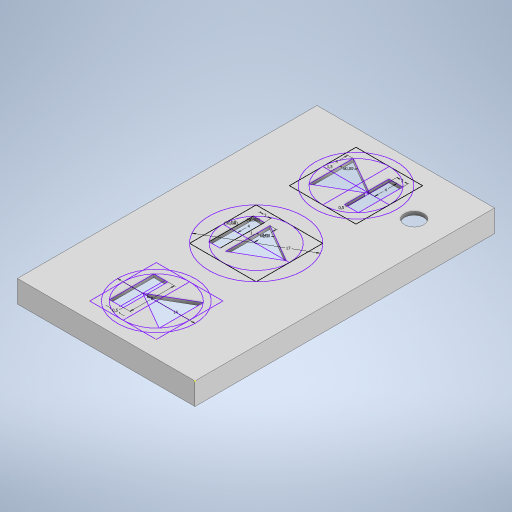
# Autodesk Inventor part: button_top
Saved by Autodesk Inventor 2024.3 (Build 283343000, 343)
## iProperties
Created: 2025-07-27
Part Number: button_top
Material: Ogólny
Document SubType Name: Modeling
Designer: User
Density: 1 g/cm^3
Appearance: Domyślna
Author: User
Autodesk Inventor part; units mm, degrees
ref_plane "YZ Plane" through (0, 0, 0) normal (1, 0, 0) x (0, 1, 0)
ref_plane "XZ Plane" through (0, 0, 0) normal (0, 1, 0) x (-1, 0, 0)
ref_plane "XY Plane" through (0, 0, 0) normal (0, 0, 1) x (1, 0, 0)
sketch "Szkic1" plane through (0, 0, 0) normal (0, 1, 0) x (-1, 0, 0)
  line L0 (0, 0) -> (32, 0)
  line L1 (32, 0) -> (32, -54)
  line L2 (32, -54) -> (0, -54)
  line L3 (0, -54) -> (0, 0)
  line L4 (32, -54) -> (32, -36)
  line L5 (32, -36) -> (0, -36)
  line L6 (32, 0) -> (32, -18)
  line L7 (32, -18) -> (0, -18)
  line L8 (32, -18) -> (32, -16)
  line L9 (32, -18) -> (32, -20)
  line L10 (32, 0) -> (32, -2)
  line L11 (32, 0) -> (32, -2)
  line L12 (32, -2) -> (0, -2)
  line L13 (0, -2) -> (0, 0)
  line L14 (0, 0) -> (32, 0)
  line L15 (32, -16) -> (32, -20)
  line L16 (32, -20) -> (0, -20)
  line L17 (0, -20) -> (0, -16)
  line L18 (0, -16) -> (32, -16)
  line L19 (32, 0) -> (32, -20)
  line L20 (32, -20) -> (30, -20)
  line L21 (30, -20) -> (30, 0)
  line L22 (30, 0) -> (32, 0)
  line L23 (0, 0) -> (0, -20)
  line L24 (0, -20) -> (2, -20)
  line L25 (2, -20) -> (2, 0)
  line L26 (2, 0) -> (0, 0)
  line L27 (16, -54) -> (16, -45)
  line L28 (16, -54) -> (25, -54) construction
  circle A0 centre (16, -45) radius 1.5
  circle A1 centre (16, -27) radius 1.5
  circle A2 centre (16, -9) radius 1.5
  line L29 (32, -20) -> (0, -20)
  line L30 (30, -38) -> (30, -18)
  line L31 (0, -34) -> (32, -34)
  line L32 (2, -38) -> (2, -18)
  line L33 (32, -38) -> (0, -38)
  line L34 (30, -56) -> (30, -36)
  line L35 (0, -52) -> (32, -52)
  line L36 (2, -56) -> (2, -36)
  line L37 (30, -2) -> (30, -1)
  line L38 (2, -2) -> (2, -1)
  line L39 (30, -2) -> (31, -2)
  line L40 (2, -16) -> (2, -17)
  line L41 (2, -17) -> (1, -17)
  line L42 (1, -17) -> (31, -17)
  line L43 (31, -17) -> (31, -1)
  line L44 (31, -1) -> (1, -1)
  line L45 (1, -1) -> (1, -17)
  line L46 (31, -35) -> (31, -19)
  line L47 (1, -35) -> (31, -35)
  line L48 (1, -19) -> (1, -35)
  line L49 (31, -19) -> (1, -19)
  line L50 (31, -53) -> (31, -37)
  line L51 (1, -53) -> (31, -53)
  line L52 (1, -37) -> (1, -53)
  line L53 (31, -37) -> (1, -37)
  line L54 (22, -39) -> (10, -39)
  line L55 (10, -39) -> (10, -51)
  line L56 (10, -51) -> (22, -51)
  line L57 (22, -51) -> (22, -39)
  line L58 (22, -39) -> (10, -51) construction
  line L59 (10, -39) -> (22, -51) construction
  line L60 (22, -21) -> (10, -21)
  line L61 (10, -21) -> (10, -33)
  line L62 (10, -33) -> (22, -33)
  line L63 (22, -33) -> (22, -21)
  line L64 (22, -21) -> (10, -33) construction
  line L65 (10, -21) -> (22, -33) construction
  line L66 (22, -3) -> (10, -3)
  line L67 (10, -3) -> (10, -15)
  line L68 (10, -15) -> (22, -15)
  line L69 (22, -15) -> (22, -3)
  line L70 (22, -3) -> (10, -15) construction
  line L71 (10, -3) -> (22, -15) construction
  circle A3 centre (16, -45) radius 6
  circle A4 centre (16, -27) radius 6
  circle A5 centre (16, -9) radius 6
  point P0 (30, -16)
  point P1 (30, -34)
  point P2 (2, -34)
  point P3 (30, -52)
  point P4 (2, -52)
  point P5 (16, 0)
  dimension "d0" = 32
  dimension "d1" = 54
  dimension "d13" = 18
  dimension "d14" = 18
  dimension "d15" = 2
  dimension "d16" = 2
  dimension "d17" = 2
  dimension "d18" = 2
  dimension "d19" = 2
  dimension "d20" = 9
  dimension "d21" = 90
  dimension "d22" = 3
  dimension "d25" = 18
  dimension "d32" = 18
  dimension "d39" = 1
  dimension "d40" = 1
  dimension "d41" = 1
  dimension "d42" = 1
  dimension "d43" = 1
  dimension "d48" = 18
  dimension "d53" = 12
  dimension "d54" = 12
  dimension "d55" = 12
  dimension "d56" = 12
  dimension "d57" = 12
  dimension "d58" = 12
  dimension "d59" = 3
  constraints: 144 end point, 18 parallel, 17 point on line, 13 perpendicular, 8 midpoint, 6 centre point, 6 horizontal, 5 vertical, 4 coincident, 3 collinear, 1 tangent, 44 other
  measures "d0" distance of L1.end L2.end
  measures "d1" distance of L0.end L1.end
  measures "d13" distance of L1.end L4.end
  measures "d14" distance of L0.end L6.end
  measures "d15" distance of L6.end L8.end
  measures "d16" distance of L6.end L9.end
  measures "d17" distance of L0.end L10.end
  measures "d18" distance of L9.end L20.end
  measures "d19" distance of L24.end L16.end
  measures "d20" distance of L27.start L27.end
  measures "d21" angle of L28 L27
  measures "d22" diameter of A0
  measures "d25" distance of A0.centre A1.centre
  measures "d32" distance of L10.end L29.start
  measures "d39" distance of L37.start L37.end
  measures "d40" distance of L38.start L38.end
  measures "d41" distance of L37.start L39.end
  measures "d42" distance of L40.start L40.end
  measures "d43" distance of L40.end L41.end
  measures "d48" distance of L42.end L46.start
  measures "d53" distance of L56.end L55.end
  measures "d54" distance of L55.end L54.end
  measures "d55" distance of L62.end L61.end
  measures "d56" distance of L61.end L60.end
  measures "d57" distance of L68.end L67.end
  measures "d58" distance between parallel lines of L66 L68
  measures "d59" distance from line of point (16, 0) L66
extrude "Wyciągnięcie proste1" add sketch "Szkic1" along normal blind 2 contours L0 L25 L44 L45 L12 L3 | L0 L21 L44 L25 | L12 L45 L18 L3 | L0 L1 L12 L43 L44 L21 | L44 L21 L12 L25 | L25 L12 L45 L44 | L18 L45 L41 L25 L7 L3 | L12 L25 L18 L45 | L44 L43 L12 L21 | L12 L21 L18 L25 | L7 L25 L49 L48 L16 L3 | L18 L25 L41 L45 | L1 L18 L43 L12 | L12 L43 L18 L21 | L18 L21 L42 L25 | L16 L48 L31 L3 | L25 L42 L21 L7 | L7 L21 L49 L25 | L1 L7 L21 L42 L43 L18 | L18 L43 L42 L21 | L31 L48 L47 L32 L5 L3 | L48 L49 L25 L16 | L16 L32 L31 L48 | L7 L1 L16 L46 L49 L21 | L49 L21 L16 L25 | L5 L32 L53 L52 L33 L3 | L31 L32 L47 L48 | L16 L30 L31 L32 | L49 L46 L16 L21 | L1 L31 L46 L16 | L33 L52 L35 L3 | L32 L47 L30 L5 | L5 L30 L53 L32 | L31 L30 L47 L32 | L16 L46 L31 L30 | L1 L5 L30 L47 L46 L31 | L35 L52 L51 L36 L2 L3 | L52 L53 L32 L33 | L33 L36 L35 L52 | L5 L1 L33 L50 L53 L30 | L53 L30 L33 L32 | L31 L46 L47 L30 | L35 L36 L51 L52 | L33 L34 L35 L36 | L53 L50 L33 L30 | L1 L35 L50 L33 | L36 L51 L27 L2 | L35 L27 L51 L36 | L33 L50 L35 L34 | L1 L2 L34 L51 L50 L35 | L27 L51 L34 L2 | L35 L34 L51 L27 | L35 L50 L51 L34
extrude "Wyciągnięcie proste3" cut sketch "Szkic1" along normal blind 1.4 contours L44 L21 L12 L25 | L25 L12 L45 L44 | L12 L25 L18 L45 | L44 L43 L12 L21 | L12 L21 L18 L25 | L18 L25 L41 L45 | L12 L43 L18 L21 | L18 L21 L42 L25 | L18 L43 L42 L21 | L48 L49 L25 L16 | L16 L32 L31 L48 | L49 L21 L16 L25 | L31 L32 L47 L48 | L16 L30 L31 L32 | L49 L46 L16 L21 | L31 L30 L47 L32 | L16 L46 L31 L30 | L52 L53 L32 L33 | L33 L36 L35 L52 | L53 L30 L33 L32 | L31 L46 L47 L30 | L35 L36 L51 L52 | L33 L34 L35 L36 | L53 L50 L33 L30 | L35 L27 L51 L36 | L33 L50 L35 L34 | L35 L34 L51 L27 | L35 L50 L51 L34
chamfer "Faza1" distance 4 angle 45 12 edges at (-31, 0.7, -1) (-31, 0.7, -17) (-1, 0.7, -17) (-1, 0.7, -1) (-31, 0.7, -35) (-31, 0.7, -19) (-1, 0.7, -19) (-1, 0.7, -35) (-1, 0.7, -37) (-31, 0.7, -37) (-31, 0.7, -53) (-1, 0.7, -53)
sketch "Szkic2" plane through (0, 2, 0) normal (0, 1, 0) x (1, 0, 0)
  line L0 (-10, 51) -> (-10, 39) projected
  line L1 (-10, 45) -> (-1, 45)
  line L2 (-1, 41) -> (-1, 49) projected
  circle A0 centre (-5.5, 45) radius 1.75
  point P0 (0, 0)
  dimension "d63" = 3.5
  constraints: 3 midpoint, 2 end point, 1 centre point
  measures "d63" diameter of A0
extrude "Wyciągnięcie proste4" cut sketch "Szkic2" against normal blind 10
move faces "Przesuń1" translate (0, -2, 0) faces at (-31.6667, 0, -22.3333)
sketch "Szkic6" plane through (0, 2, 0) normal (0, 1, 0) x (1, 0, 0)
  line L0 (-22, 51) -> (-10, 51) projected
  line L1 (-10, 51) -> (-10, 39) projected
  line L2 (-22, 51) -> (-10, 51)
  line L3 (-10, 51) -> (-10, 39)
  line L4 (-10, 39) -> (-22, 39)
  line L5 (-22, 39) -> (-22, 51)
  line L6 (-22, 33) -> (-10, 33) projected
  line L7 (-10, 33) -> (-10, 21) projected
  line L8 (-22, 33) -> (-10, 33)
  line L9 (-10, 33) -> (-10, 21)
  line L10 (-10, 21) -> (-22, 21)
  line L11 (-22, 21) -> (-22, 33)
  circle A0 centre (-16, 27) radius 6
  circle A1 centre (-16, 45) radius 6
  line L12 (-22, 45) -> (-10, 45)
  line L13 (-16, 51) -> (-16, 39)
  line L14 (-22, 45) -> (-20.5, 45)
  line L15 (-20.5, 45) -> (-20.5, 49)
  line L16 (-20.5, 49) -> (-13.5718, 45)
  line L17 (-13.5718, 45) -> (-13.5718, 49)
  line L18 (-13.5718, 49) -> (-11.5718, 49)
  line L19 (-11.5718, 49) -> (-11.5718, 45)
  line L20 (-16, 39) -> (-16, 51)
  line L21 (-20.5, 45) -> (-20.5, 41)
  line L22 (-20.5, 41) -> (-13.5718, 45)
  line L23 (-13.5718, 45) -> (-13.5718, 41)
  line L24 (-13.5718, 41) -> (-11.5718, 41)
  line L25 (-11.5718, 41) -> (-11.5718, 45)
  line L26 (-22, 27) -> (-10, 27)
  line L27 (-22, 27) -> (-20.5, 27)
  line L28 (-20.5, 27) -> (-20.5, 31)
  line L29 (-20.5, 31) -> (-18.5, 31)
  line L30 (-18.5, 31) -> (-18.5, 27)
  line L31 (-18.5, 27) -> (-17.5, 27)
  line L32 (-17.5, 27) -> (-17.5, 31)
  line L33 (-17.5, 31) -> (-10.5718, 27)
  circle A2 centre (-16, 27) radius 6
  line L34 (-20.5, 27) -> (-20.5, 23)
  line L35 (-20.5, 23) -> (-18.5, 23)
  line L36 (-18.5, 23) -> (-18.5, 27)
  line L37 (-17.5, 27) -> (-17.5, 23)
  line L38 (-17.5, 23) -> (-10.5718, 27)
  line L39 (-22, 39) -> (-10, 39)
  line L40 (-10, 39) -> (-10, 51)
  line L41 (-10, 51) -> (-22, 51)
  line L42 (-22, 51) -> (-22, 39)
  line L43 (-10, 15) -> (-22, 15)
  line L44 (-22, 15) -> (-22, 3)
  line L45 (-10, 15) -> (-22, 15)
  line L46 (-22, 15) -> (-22, 3)
  line L47 (-22, 3) -> (-10, 3)
  line L48 (-10, 3) -> (-10, 15)
  circle A3 centre (-16, 9) radius 6
  line L49 (-10, 9) -> (-22, 9)
  line L50 (-16, 15) -> (-16, 3)
  line L51 (-10, 9) -> (-11.5, 9)
  line L52 (-11.5, 9) -> (-11.5, 13)
  line L53 (-11.5, 13) -> (-18.4282, 9)
  line L54 (-18.4282, 9) -> (-18.4282, 13)
  line L55 (-18.4282, 13) -> (-20.4282, 13)
  line L56 (-20.4282, 13) -> (-20.4282, 9)
  line L57 (-18.4282, 9) -> (-18.4282, 5)
  line L58 (-11.5, 9) -> (-11.5, 5)
  line L59 (-11.5, 5) -> (-18.4282, 9)
  line L60 (-16, 3) -> (-16, 15)
  line L61 (-20.4282, 5) -> (-20.4282, 9)
  line L62 (-18.4282, 5) -> (-20.4282, 5)
  line L63 (-10, 3) -> (-22, 3)
  line L64 (-22, 3) -> (-22, 15)
  line L65 (-22, 15) -> (-10, 15)
  line L66 (-10, 15) -> (-10, 3)
  circle A4 centre (-16, 45) radius 7.3724
  circle A5 centre (-16, 27) radius 8.5
  circle A6 centre (-16, 9) radius 7
  line L67 (-13.5718, 49) -> (-14.0718, 49)
  line L68 (-14.0718, 49) -> (-14.0718, 41)
  line L69 (-14.0718, 41) -> (-13.5718, 41)
  line L70 (-13.5718, 41) -> (-13.5718, 49)
  line L71 (-18.4282, 13) -> (-17.9282, 13)
  line L72 (-17.9282, 13) -> (-17.9282, 5)
  line L73 (-17.9282, 5) -> (-18.4282, 5)
  line L74 (-18.4282, 5) -> (-18.4282, 13)
  point P0 (0, 0)
  point P1 (-10, 3)
  point P2 (-22, 3)
  point P3 (-20.5, 41.0314)
  point P4 (-20.5, 48.9686)
  point P5 (-20.4816, 41.0106)
  point P6 (-20.4816, 48.9894)
  point P7 (-20.5, 23.0314)
  point P8 (-20.5, 30.9686)
  point P9 (-20.4721, 31)
  point P10 (-20.4721, 23)
  point P11 (-11.5, 12.9686)
  point P12 (-11.5, 5.0314)
  point P13 (-11.5184, 12.9894)
  point P14 (-11.5184, 5.0106)
  point P15 (-14.0718, 44.7113)
  point P16 (-14.0718, 45.2887)
  point P17 (-17.9282, 9.2887)
  point P18 (-17.9282, 8.7113)
  dimension "d101" = 1.5
  dimension "d102" = 4
  dimension "d103" = 60
  dimension "d104" = 4
  dimension "d105" = 2
  dimension "d106" = 1.5
  dimension "d107" = 4
  dimension "d108" = 90
  dimension "d109" = 2
  dimension "d110" = 90
  dimension "d111" = 1
  dimension "d112" = 4
  dimension "d113" = 60
  dimension "d118" = 17
  dimension "d119" = 14
  dimension "d120" = 0.5
  dimension "d121" = 0.5
  dimension "d122" = 8
  constraints: 142 end point, 12 point on line, 11 parallel, 10 midpoint, 10 perpendicular, 10 point on circle, 8 symmetric about line, 7 centre point, 5 horizontal, 3 coincident, 1 tangent, 1 vertical, 1 other
  measures "d101" distance of L12.start L14.end
  measures "d102" distance of L14.end L15.end
  measures "d103" angle of L15 L16
  measures "d104" distance of L16.end L17.end
  measures "d105" distance of L17.end L18.end
  measures "d106" distance of L26.start L27.end
  measures "d107" distance of L27.end L28.end
  measures "d108" angle of L28 L27
  measures "d109" distance of L28.end L29.end
  measures "d110" angle of L28 L29
  measures "d111" distance of L30.end L31.end
  measures "d112" distance of L31.end L32.end
  measures "d113" angle of L32 L33
  measures "d118" diameter of A5
  measures "d119" diameter of A6
  measures "d120" distance of L69.end L68.end
  measures "d121" distance of L72.end L73.end
  measures "d122" distance of L71.end L72.end
extrude "Wyciągnięcie proste7" add sketch "Szkic6" against normal up to surface (0.6 mm away) contours L0 A4 L5 | L0 A1 L16 L15 L5 A4 | L0 A4 L1 A1 | L13 L16 A1 | A1 L12 L19 L18 L67 L68 L16 L13 | L0 L1 A4 | A1 L21 L22 L4 A4 L5 | L12 L21 A1 | A1 L15 L12 | A4 L4 L5 | L1 A4 L4 A1 | A1 L13 L22 L68 L69 L24 L25 L12 | L1 L4 A4 | A1 L22 L13 | L6 A0 L29 L28 L11 | L6 L7 A0 | A0 L26 L33 L32 L30 L29 | A0 L34 L35 L10 L11 | L26 L34 A0 | A0 L28 L26 | L7 L10 A0 | A0 L35 L36 L26 L37 L38 | L48 A6 L43 | A6 L48 A3 L52 L53 L43 | A3 L44 A6 L43 | L50 L53 L72 L71 L55 L56 L49 A3 | A3 L53 L50 | A6 L44 L43 | L49 L52 A3 | L48 A6 L47 A3 L59 L58 | A3 L58 L49 | A3 L47 A6 L44 | L49 L61 L62 L73 L72 L59 L50 A3 | L48 L47 A6 | A6 L47 L44 | L50 L59 A3
